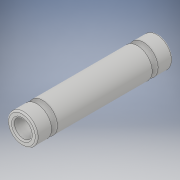
# Autodesk Inventor part: Component 12 (Piston Axis)
Saved by Autodesk Inventor 2018 (Build 220112000, 112)
## iProperties
Created: 2023-03-14
Part Number: Component 12 (Piston Axis)
Material: Generic
Document SubType Name: Modeling
Designer: Habib Mohamed
Density: 1 g/cm^3
Appearance: Default
Author: Habib Mohamed
Autodesk Inventor part; units mm, degrees
ref_plane "YZ Plane" through (0, 0, 0) normal (1, 0, 0) x (0, 1, 0)
ref_plane "XZ Plane" through (0, 0, 0) normal (0, 1, 0) x (-1, 0, 0)
ref_plane "XY Plane" through (0, 0, 0) normal (0, 0, 1) x (1, 0, 0)
sketch "Sketch1" plane through (0, 0, 0) normal (1, 0, 0) x (0, 1, 0)
  line L0 (0, 0) -> (0, -27.6453) construction
  line L1 (1.5, 0) -> (1.5, -11.5)
  line L2 (2.25, 0) -> (1.5, 0)
  arc A0 (2.5, -2.5) -> (2.5, -3.5) centre (2.5, -3) ccw
  line L3 (0, 0) -> (10.0223, 0) construction
  arc A1 (2.5, -0.25) -> (2.25, 0) centre (2.25, -0.25) ccw
  line L4 (2.5, -11.5) -> (2.5, -3.5)
  line L5 (2.5, -2.5) -> (2.5, -0.25)
  line L6 (1.5, -11.5) -> (14.7413, -11.5) construction
  line L7 (0, -23) -> (0, 4.6453) construction
  line L8 (1.5, -23) -> (1.5, -11.5)
  line L9 (2.25, -23) -> (1.5, -23)
  arc A2 (2.5, -19.5) -> (2.5, -20.5) centre (2.5, -20) ccw
  line L10 (0, -23) -> (10.0223, -23) construction
  arc A3 (2.25, -23) -> (2.5, -22.75) centre (2.25, -22.75) ccw
  line L11 (2.5, -11.5) -> (2.5, -19.5)
  line L12 (2.5, -20.5) -> (2.5, -22.75)
  point P0 (2.5, 0)
  point P1 (1.875, 0)
  point P2 (2.5, -23)
  dimension "d2" = 1.5
  dimension "d3" = 3
  dimension "d4" = 1
  dimension "d5" = 0.25
  dimension "d6" = 2.25
  dimension "d7" = 1
  dimension "d8" = 23
  constraints: 26 end point, 11 symmetric about line, 8 point on circle, 4 centre point, 4 point on line, 3 tangent, 2 horizontal, 2 perpendicular, 2 vertical, 1 midpoint, 2 other
  measures "d2" distance between parallel lines of L1 L0
  measures "d3" distance from line of L2 A0.centre
  measures "d4" diameter of A0
  measures "d5" radius of A1
  measures "d6" distance of L5.start L5.end
  measures "d7" distance between parallel lines of L1 L5
  measures "d8" distance of L1.start L8.start
revolve "Revolution1" add sketch "Sketch1" angle 360 about axis through (0, 0, -23) along (0, 0, 1)
fillet "Fillet1" radius 0.25 2 edges at (0, -1.5, 0) (0, -1.5, -23)
body "Solid1"
